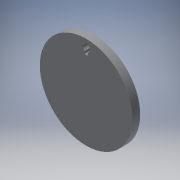
# Autodesk Inventor part: Circular Pattern
Saved by Autodesk Inventor 2019 Beta2 (Build 230110000, 110) ContinuousBuild 0
## iProperties
Created: 2013-12-15
Part Number: Circular Pattern
Material: Generic
Document SubType Name: Modeling
Designer: John
Density: 1 g/cm^3
Appearance: Default
Author: John
Autodesk Inventor part; units mm, degrees
ref_plane "YZ Plane" through (0, 0, 0) normal (1, 0, 0) x (0, 1, 0)
ref_plane "XZ Plane" through (0, 0, 0) normal (0, 1, 0) x (-1, 0, 0)
ref_plane "XY Plane" through (0, 0, 0) normal (0, 0, 1) x (1, 0, 0)
sketch "Sketch1" plane through (0, 0, 0) normal (0, 0, 1) x (1, 0, 0)
  circle A0 centre (0, 0) radius 38.1
  dimension "d0" = 76.2
  constraints: 1 centre point, 1 coincident
  measures "d0" diameter of A0
extrude "Extrusion1" add sketch "Sketch1" along normal blind 6.35
sketch "Sketch2" plane through (0, 0, 6.35) normal (0, 0, 1) x (1, 0, 0)
  circle A0 centre (0, 0) radius 38.1 projected
  circle A1 centre (0, 31.75) radius 3.175
  dimension "d3" = 6.35
  dimension "d6" = 31.75
  constraints: 1 centre point, 1 vertical alignment
  measures "d3" diameter of A1
  measures "d6" distance of A0.centre A1.centre
extrude "Extrusion2" cut sketch "Sketch2" against normal through all contours A1
sketch "Sketch3" plane through (0, 0, 6.35) normal (0, 0, 1) x (1, 0, 0)
  circle A0 centre (0, 31.75) radius 3.175 projected
  line L0 (0, 31.75) -> (1.27, 31.75)
  line L1 (1.27, 31.75) -> (1.27, 26.67)
  line L2 (1.27, 26.67) -> (0, 26.67)
  line L3 (0, 26.67) -> (0, 31.75)
  line L4 (0, 31.75) -> (-1.27, 31.75)
  line L5 (-1.27, 31.75) -> (-1.27, 26.67)
  line L6 (-1.27, 26.67) -> (0, 26.67)
  line L7 (0, 26.67) -> (0, 31.75)
  dimension "d9" = 1.27
  dimension "d10" = 5.08
  constraints: 16 end point, 4 parallel, 2 equal length, 2 horizontal, 2 perpendicular
  measures "d9" distance of L1.end L2.end
  measures "d10" distance of L0.end L1.end
extrude "Extrusion3" cut sketch "Sketch3" against normal through all contours L5 L4 L3 A0 | A0 L3 L6 L5 | L1 L2 L3 A0 | A0 L3 L0 L1
body "Solid1"
